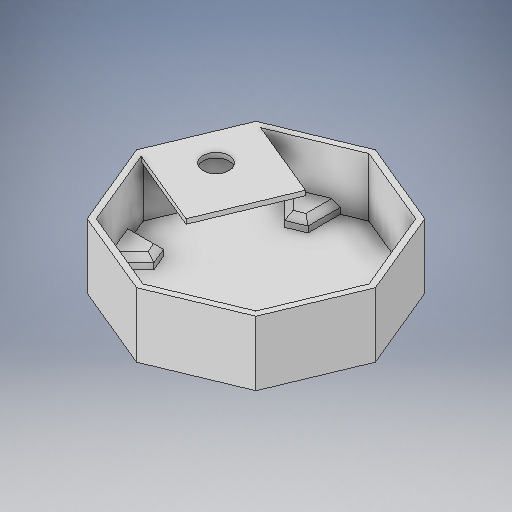
# Autodesk Inventor part: BaseHex
Saved by Autodesk Inventor 2025.2 (Build 292293000, 293)
## iProperties
Created: 2025-04-01
Part Number: BaseHex
Material: Generic
Document SubType Name: Modeling
Designer: Tiago
Density: 1 g/cm^3
Appearance: Default
Author: Tiago
Autodesk Inventor part; units mm, degrees
ref_plane "YZ Plane" through (0, 0, 0) normal (1, 0, 0) x (0, 1, 0)
ref_plane "XZ Plane" through (0, 0, 0) normal (0, 1, 0) x (-1, 0, 0)
ref_plane "XY Plane" through (0, 0, 0) normal (0, 0, 1) x (1, 0, 0)
sketch "Sketch1" plane through (0, 0, 0) normal (0, 0, 1) x (1, 0, 0)
  circle A0 centre (0, 0) radius 100
  line L0 (100, 0) -> (70.7107, -70.7107)
  line L1 (70.7107, -70.7107) -> (0, -100)
  line L2 (0, -100) -> (-70.7107, -70.7107)
  line L3 (-70.7107, -70.7107) -> (-100, 0)
  line L4 (-100, 0) -> (-70.7107, 70.7107)
  line L5 (-70.7107, 70.7107) -> (0, 100)
  line L6 (0, 100) -> (70.7107, 70.7107)
  line L7 (70.7107, 70.7107) -> (100, 0)
  line L8 (0, 94.588) -> (-66.8838, 66.8838)
  line L9 (-66.8838, 66.8838) -> (-94.588, 0)
  line L10 (-94.588, 0) -> (-66.8838, -66.8838)
  line L11 (-66.8838, -66.8838) -> (0, -94.588)
  line L12 (0, -94.588) -> (66.8838, -66.8838)
  line L13 (66.8838, -66.8838) -> (94.588, 0)
  line L14 (94.588, 0) -> (66.8838, 66.8838)
  line L15 (66.8838, 66.8838) -> (0, 94.588)
  line L16 (-28.6155, 28.6155) -> (0, 40.4684)
  line L17 (28.6155, 28.6155) -> (40.4684, 0)
  line L18 (28.6155, -28.6155) -> (0, -40.4684)
  line L19 (-28.6155, -28.6155) -> (-40.4684, 0)
  line L20 (0, -40.4684) -> (0, -94.588)
  line L21 (28.6155, -28.6155) -> (66.8838, -66.8838)
  line L22 (40.4684, 0) -> (94.588, 0)
  line L23 (-40.4684, 0) -> (-94.588, 0)
  line L24 (-28.6155, -28.6155) -> (-66.8838, -66.8838)
  line L25 (28.6155, 28.6155) -> (66.8838, 66.8838)
  line L26 (0, 40.4684) -> (0, 94.588)
  line L27 (-28.6155, 28.6155) -> (-66.8838, 66.8838)
  line L28 (16.9457, -60.5091) -> (26.5128, -83.6061)
  line L29 (30.8039, -54.7688) -> (40.371, -77.8658)
  line L30 (16.9457, -60.5091) -> (30.8039, -54.7688)
  line L31 (16.9457, -60.5091) -> (16.9457, -87.5689)
  line L32 (30.8039, -54.7688) -> (49.9381, -73.903)
  line L33 (60.5091, 16.9457) -> (87.5689, 16.9457)
  line L34 (60.5091, 16.9457) -> (83.6061, 26.5128)
  line L35 (60.5091, 16.9457) -> (54.7688, 30.8039)
  line L36 (54.7688, 30.8039) -> (73.903, 49.9381)
  line L37 (54.7688, 30.8039) -> (77.8658, 40.371)
  line L38 (-16.9457, 60.5091) -> (-16.9457, 87.5689)
  line L39 (-16.9457, 60.5091) -> (-26.5128, 83.6061)
  line L40 (-16.9457, 60.5091) -> (-30.8039, 54.7688)
  line L41 (-30.8039, 54.7688) -> (-49.9381, 73.903)
  line L42 (-30.8039, 54.7688) -> (-40.371, 77.8658)
  line L43 (-60.5091, -16.9457) -> (-87.5689, -16.9457)
  line L44 (-60.5091, -16.9457) -> (-83.6061, -26.5128)
  line L45 (-60.5091, -16.9457) -> (-54.7688, -30.8039)
  line L46 (-54.7688, -30.8039) -> (-73.903, -49.9381)
  line L47 (-54.7688, -30.8039) -> (-77.8658, -40.371)
  dimension "d0" = 200
  dimension "d1" = 5
  dimension "d13" = 360
  constraints: 96 end point, 3 point on line, 2 vertical, 1 coincident, 1 collinear, 1 horizontal, 1 horizontal alignment, 1 perpendicular, 54 other
  measures "d1" distance between parallel lines of L5 L8
extrude "Extrusion1" add sketch "Sketch1" along normal blind 50 contours L0 L1 L2 L3 L4 L5 L6 L7
extrude "Extrusion2" add sketch "Sketch1" against normal blind 5 contours L0 L1 L2 L3 L4 L5 L6 L7 | L26 L16 L27 L8 L41 L40 L38 | L15 L25 L17 L22 L13 L21 L18 L20 L11 L24 L19 L23 L9 L27 L16 L26 | L38 L39 L8 | L14 L36 L35 L33 L22 L17 L25 | L39 L40 L42 L8 | L14 L37 L36 | L42 L41 L8 | L14 L34 L35 L37 | L14 L33 L34 | L23 L19 L24 L10 L46 L45 L43 | L12 L32 L30 L31 L20 L18 L21 | L43 L44 L10 | L12 L29 L32 | L44 L45 L47 L10 | L12 L28 L30 L29 | L47 L46 L10 | L12 L31 L28
extrude "Extrusion3" add sketch "Sketch1" along normal blind 10 contours L38 L39 L8 | L39 L40 L42 L8 | L14 L37 L36 | L42 L41 L8 | L14 L34 L35 L37 | L14 L33 L34 | L43 L44 L10 | L12 L29 L32 | L44 L45 L47 L10 | L12 L28 L30 L29 | L47 L46 L10 | L12 L31 L28
chamfer "Chamfer1" distance 5 angle 45 12 edges at (64.3359, 40.371, 10) (74.039, 16.9457, 10) (57.639, 23.8748, 10) (23.8748, -57.639, 10) (16.9457, -74.039, 10) (40.371, -64.3359, 10) (-64.3359, -40.371, 10) (-57.639, -23.8748, 10) (-74.039, -16.9457, 10) (-40.371, 64.3359, 10) (-23.8748, 57.639, 10) (-16.9457, 74.039, 10)
sketch "Sketch3" plane through (0, 0, 50) normal (0, 0, 1) x (1, 0, 0)
  line L0 (-70.7107, 70.7107) -> (-100, 0) projected
  circle A0 centre (0, 0) radius 100
  line L1 (-100, 0) -> (-70.7107, -70.7107) projected
  line L2 (-100, 0) -> (-70.7107, 70.7107)
  line L3 (-70.7107, 70.7107) -> (0, 100)
  line L4 (0, 100) -> (70.7107, 70.7107)
  line L5 (70.7107, 70.7107) -> (100, 0)
  line L6 (100, 0) -> (70.7107, -70.7107)
  line L7 (70.7107, -70.7107) -> (0, -100)
  line L8 (0, -100) -> (-70.7107, -70.7107)
  line L9 (-70.7107, -70.7107) -> (-100, 0)
  circle A1 centre (0, 0) radius 5
  line L10 (-66.8838, -66.8838) -> (0, -94.588)
  line L11 (0, -94.588) -> (66.8838, -66.8838)
  line L12 (66.8838, -66.8838) -> (94.588, 0)
  line L13 (94.588, 0) -> (66.8838, 66.8838)
  line L14 (66.8838, 66.8838) -> (0, 94.588)
  line L15 (0, 94.588) -> (-66.8838, 66.8838)
  line L16 (-66.8838, 66.8838) -> (-94.588, 0)
  line L17 (-94.588, 0) -> (-66.8838, -66.8838)
  dimension "d30" = 10
  constraints: 32 end point, 3 coincident, 2 centre point, 1 point on circle, 24 other
  measures "d30" diameter of A1
extrude "Extrusion5" cut sketch "Sketch3" against normal blind 5 contours L3 L4 L5 L6 L7 L8 L1 L0
sketch "Sketch4" plane through (0, 0, 45) normal (0, 0, 1) x (1, 0, 0)
  line L0 (-70.7107, -70.7107) -> (-41.4258, -0.0106)
  line L1 (0, 100) -> (70.7107, 70.7107) projected
  line L2 (70.7107, -70.7107) -> (0, -100) projected
  line L3 (0, -100) -> (40.3895, -2.4912)
  line L4 (0, -100) -> (-70.7107, -70.7107) projected
  line L5 (-41.4258, -0.0106) -> (29.2849, -29.2999)
  circle A0 centre (-23.6574, -57.114) radius 11
  line L6 (0, -100) -> (-70.7107, -70.7107)
  line L7 (-70.7107, -70.7107) -> (-100, 0)
  line L8 (-100, 0) -> (-70.7107, 70.7107)
  line L9 (-70.7107, 70.7107) -> (0, 100)
  line L10 (0, 100) -> (70.7107, 70.7107)
  line L11 (70.7107, 70.7107) -> (100, 0)
  line L12 (100, 0) -> (70.7107, -70.7107)
  line L13 (70.7107, -70.7107) -> (0, -100)
  line L14 (0, -94.588) -> (-66.8838, -66.8838) projected
  line L15 (0, -94.588) -> (-66.8838, -66.8838)
  line L16 (-66.8838, -66.8838) -> (-94.588, 0)
  line L17 (-94.588, 0) -> (-66.8838, 66.8838)
  line L18 (-66.8838, 66.8838) -> (0, 94.588)
  line L19 (0, 94.588) -> (66.8838, 66.8838)
  line L20 (66.8838, 66.8838) -> (94.588, 0)
  line L21 (94.588, 0) -> (66.8838, -66.8838)
  line L22 (66.8838, -66.8838) -> (0, -94.588)
  line L23 (-33.4419, -80.7359) -> (-23.6574, -57.114)
  point P0 (0, 0)
  point P1 (0, 0)
  point P2 (0, 0)
  point P3 (-68.0047, -64.1779)
  point P4 (2.706, -93.4672)
  dimension "d33" = 22
  constraints: 40 end point, 3 perpendicular, 2 coincident, 1 centre point, 1 midpoint, 1 point on line, 34 other
  measures "d33" diameter of A0
extrude "Extrusion6" add sketch "Sketch4" along normal blind 4 contours L7 L8 L9 L1 L11 L12 L2 L3 L22 L21 L20 L19 L18 L17 L16 L0 | L0 L16 L14 L22 L3 L4 | L0 L5 L3 L22 L14 L16
body "Solid1"
